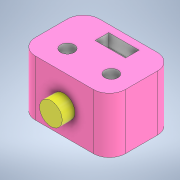
# Autodesk Inventor part: finalface4
Saved by Autodesk Inventor 2021 (Build 250183000, 183)
## iProperties
Created: 2021-07-12
Part Number: finalface4
Material: Generic
Document SubType Name: Modeling
Designer: Dell
Density: 1 g/cm^3
Appearance: Default
Author: Dell
Autodesk Inventor part; units mm, degrees
ref_plane "YZ Plane" through (0, 0, 0) normal (1, 0, 0) x (0, 1, 0)
ref_plane "XZ Plane" through (0, 0, 0) normal (0, 1, 0) x (-1, 0, 0)
ref_plane "XY Plane" through (0, 0, 0) normal (0, 0, 1) x (1, 0, 0)
sketch "Sketch1" plane through (0, 0, 0) normal (0, 0, 1) x (1, 0, 0)
  line L0 (0, 0) -> (-17.8576, 0)
  line L1 (-17.8576, 0) -> (-17.8576, 11.024)
  line L2 (-17.8576, 11.024) -> (0, 11.024)
  line L3 (0, 11.024) -> (0, 0)
  constraints: 8 end point, 2 parallel, 1 horizontal, 1 perpendicular
extrude "Extrusion1" add sketch "Sketch1" along normal blind 12.7
sketch "Sketch2" plane through (-17.8576, 11.024, 0) normal (0, 1, 0) x (1, 0, 0)
  circle A0 centre (13.7961, -8.2519) radius 1.3228
  circle A1 centre (5.0929, -8.2519) radius 1.3477
  line L0 (12.4733, -4.1259) -> (6.4406, -4.1259)
  line L1 (6.4406, -4.1259) -> (6.4406, -1.4183)
  line L2 (6.4406, -1.4183) -> (12.4733, -1.4183)
  line L3 (12.4733, -1.4183) -> (12.4733, -4.1259)
  point P0 (17.8576, 0)
  constraints: 8 end point, 2 centre point, 2 parallel, 1 horizontal, 1 perpendicular
extrude "Extrusion2" cut sketch "Sketch2" against normal blind 2.54
fillet "Fillet1" radius 3.175 1 edges at (-17.8576, 5.512, 12.7)
fillet "Fillet2" radius 3.175 1 edges at (-17.8576, 5.512, 0)
fillet "Fillet3" radius 3.175 1 edges at (0, 5.512, 12.7)
fillet "Fillet4" radius 3.175 1 edges at (0, 5.512, 0)
sketch "Sketch3" plane through (0, 0, 0) normal (0, 0, -1) x (-1, 0, 0)
  circle A0 centre (8.0161, 5.0375) radius 2.5669
  point P0 (0, 0)
  constraints: 1 centre point
extrude "Extrusion3" cut sketch "Sketch3" against normal blind 7.62
sketch "Sketch4" plane through (0, 0, 12.7) normal (0, 0, 1) x (1, 0, 0)
  circle A0 centre (-9.0674, 5.2127) radius 2.2357
  point P0 (0, 0)
  constraints: 1 centre point
extrude "Extrusion4" add sketch "Sketch4" along normal blind 2.54
body "Solid1"
